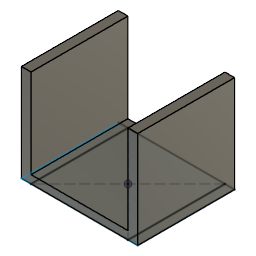
arm holder (Autodesk Fusion 360 design; units mm, degrees)
part number: 2026-08-05-14-50-43-195
Autodesk Fusion 360 part; units mm, degrees
sketch "Sketch1" plane through (0, 0, 0) normal (0, 0, 1) x (1, 0, 0)
  line L0 (38.1, 38.1) -> (-38.1, 38.1)
  line L1 (-38.1, 38.1) -> (-38.1, -38.1)
  line L2 (-38.1, -38.1) -> (38.1, -38.1)
  line L3 (38.1, -38.1) -> (38.1, 38.1)
  line L4 (38.1, 38.1) -> (-38.1, -38.1) construction
  line L5 (-38.1, 38.1) -> (38.1, -38.1) construction
  line L6 (-38.1, 38.1) -> (-45.72, 38.1)
  line L7 (-45.72, 38.1) -> (-45.72, -38.1)
  line L8 (-45.72, -38.1) -> (-38.1, -38.1)
  line L9 (-38.1, -38.1) -> (-38.1, 38.1)
  line L10 (38.1, 38.1) -> (45.72, 38.1)
  line L11 (45.72, 38.1) -> (45.72, -38.1)
  line L12 (45.72, -38.1) -> (38.1, -38.1)
  line L13 (38.1, -38.1) -> (38.1, 38.1)
  dimension "d1" = 76.2
  dimension "d2" = 76.2
  dimension "d3" = 7.62
  constraint horizontal L0
  constraint perpendicular L0 L1
  constraint parallel L0 L2
  constraint parallel L1 L3
  constraint coincident L4 origin
  constraint coincident L5 origin
  constraint horizontal L6
  constraint vertical L7
  constraint horizontal L8
  constraint vertical L9
  constraint horizontal L10
  constraint vertical L11
  constraint horizontal L12
  constraint vertical L13
  measures "d1" distance of L1.end L2.end
  measures "d2" distance of L0.end L1.end
  measures "d3" distance of L0.start L10.end
extrude "Extrude1" add sketch "Sketch1" along normal blind 6.35 contours L0 L1 L2 L3 L9 L13
sketch "Sketch2" plane through (0, 0, 0) normal (0, 0, 1) x (1, 0, 0)
extrude "Extrude2" add sketch "Sketch1" along normal blind 76.2 contours L3 L10 L11 L12 L13 | L1 L6 L7 L8 L9
